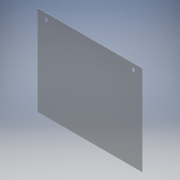
# Autodesk Inventor part: PlexiglassWall3ft
Saved by Autodesk Inventor 2017 (Build 210142000, 142)
## iProperties
Created: 2017-06-28
Part Number: PlexiglassWall3ft
Material: Generic
Document SubType Name: Modeling
Designer: sensor
Density: 1 g/cm^3
Appearance: Clear
Author: sensor
Autodesk Inventor part; units mm, degrees
ref_plane "YZ Plane" through (0, 0, 0) normal (1, 0, 0) x (0, 1, 0)
ref_plane "XZ Plane" through (0, 0, 0) normal (0, 1, 0) x (-1, 0, 0)
ref_plane "XY Plane" through (0, 0, 0) normal (0, 0, 1) x (1, 0, 0)
sketch "Sketch1" plane through (0, 0, 0) normal (0, 0, 1) x (1, 0, 0)
  line L0 (0, 0) -> (914.4, 0)
  line L1 (914.4, 0) -> (914.4, 787.4)
  line L2 (914.4, 787.4) -> (0, 787.4)
  line L3 (0, 787.4) -> (0, 0)
  circle A0 centre (76.2, 736.6) radius 12.7
  circle A1 centre (838.2, 736.6) radius 12.7011
  circle A2 centre (76.2, 749.3) radius 6.35
  circle A3 centre (838.0337, 749.3) radius 6.35
  dimension "d21" = 25.4022
  dimension "d0" = 914.4
  dimension "d1" = 787.4
  dimension "d2" = 25.4
  dimension "d5" = 50.8
  dimension "d7" = 76.2
  dimension "d11" = 12.7
  dimension "d12" = 38.1
  dimension "d17" = 38.1
  dimension "d18" = 76.2
  dimension "d19" = 50.8
  dimension "d20" = 12.7
  constraints: 8 end point, 3 centre point, 2 parallel, 1 horizontal, 1 perpendicular, 3 other
  measures "d0" distance of L1.end L2.end
  measures "d1" distance of L0.end L1.end
  measures "d2" diameter of A0
  measures "d5" distance from line of L2 A0.centre
  measures "d7" distance from line of L3 A0.centre
  measures "d11" diameter of A2
  measures "d12" distance from line of L2 A2.centre
  measures "d17" distance from line of L2 A3.centre
  measures "d18" distance from line of L1 point (838.2, 736.6)
  measures "d19" distance from line of L2 point (838.2, 736.6)
  measures "d20" diameter of A3
extrude "Extrusion2" add sketch "Sketch1" along normal blind 2.3622
body "Solid2"
